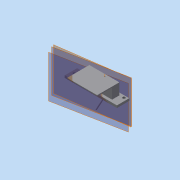
# Autodesk Inventor part: 00_TI_DLP_2000_Chip
Saved by Autodesk Inventor 2019.4 (Build 234330000, 330)
## iProperties
Created: 2019-08-06
Part Number: 00_TI_DLP_2000_Chip
Material: Generic
Document SubType Name: Modeling
Designer: diederichbenedict
Density: 1 g/cm^3
Appearance: Default
Author: diederichbenedict
Autodesk Inventor part; units mm, degrees
ref_plane "YZ Plane" through (0, 0, 0) normal (1, 0, 0) x (0, 1, 0)
ref_plane "XZ Plane" through (0, 0, 0) normal (0, 1, 0) x (-1, 0, 0)
ref_plane "XY Plane" through (0, 0, 0) normal (0, 0, 1) x (1, 0, 0)
sketch "Sketch1" plane through (0, 0, 0) normal (0, 1, 0) x (-1, 0, 0)
  line L0 (14.75, 3.5) -> (-14.75, 3.5)
  line L1 (-14.75, 3.5) -> (-14.75, -3.5)
  line L2 (-14.75, -3.5) -> (14.75, -3.5)
  line L3 (14.75, -3.5) -> (14.75, 3.5)
  line L4 (14.75, 3.5) -> (-14.75, -3.5) construction
  line L5 (-14.75, 3.5) -> (14.75, -3.5) construction
  circle A0 centre (-13, -2.25) radius 0.75
  circle A1 centre (13, -0.25) radius 0.75
  point P0 (0, 0)
  dimension "d0" = 29.5
  dimension "d1" = 7
  dimension "d2" = 1.5
  dimension "d3" = 1.5
  dimension "d4" = 5.75
  dimension "d5" = 3.75
  dimension "d6" = 1.75
  dimension "d7" = 1.75
  constraints: 12 end point, 2 centre point, 2 midpoint, 2 parallel, 1 horizontal, 1 perpendicular
  measures "d0" distance of L2.end L1.end
  measures "d1" distance of L1.end L0.end
  measures "d2" diameter of A0
  measures "d3" diameter of A1
  measures "d4" distance from line of A0.centre L0
  measures "d5" distance from line of A1.centre L0
  measures "d6" distance from line of A1.centre L3
  measures "d7" distance from line of L1 A0.centre
extrude "Extrusion1" add sketch "Sketch1" along normal blind 1.3
sketch "Sketch2" plane through (0, 0, 0) normal (0, -1, 0) x (1, 0, 0)
  line L0 (-3.64, 1.57) -> (10.48, 1.57)
  line L1 (10.48, 1.57) -> (10.48, -3.4)
  line L2 (10.48, -3.4) -> (-3.64, -3.4)
  line L3 (-3.64, -3.4) -> (-3.64, 1.57)
  line L4 (14.75, 3.5) -> (14.75, -3.5) projected
  line L5 (-14.75, -3.5) -> (-14.75, 3.5) projected
  line L6 (14.75, -3.5) -> (-14.75, -3.5) projected
  line L7 (-3.64, 0.335) -> (-2.84, 0.335)
  line L8 (-2.84, 0.335) -> (-2.84, -2.165)
  line L9 (-2.84, -2.165) -> (-3.64, -2.165)
  line L10 (-3.64, -2.165) -> (-3.64, 0.335)
  line L11 (10.48, 0.7644) -> (9.304, -0.4116)
  line L12 (10.48, 0.7644) -> (12.1431, 0.7644) construction
  line L13 (9.304, -0.4116) -> (9.304, -1.4116)
  line L14 (10.48, -2.5876) -> (9.304, -1.4116)
  line L15 (10.48, -2.5876) -> (12.1431, -2.5876) construction
  point P0 (0, 0)
  dimension "d10" = 14.12
  dimension "d11" = 4.97
  dimension "d13" = 11.11
  dimension "d14" = 0.1
  dimension "d15" = 2.5
  dimension "d16" = 0.8
  dimension "d17" = 1.235
  dimension "d18" = 135
  dimension "d19" = 135
  dimension "d20" = 1.176
  dimension "d21" = 1
  constraints: 26 end point, 4 horizontal, 4 parallel, 3 point on line, 2 equal length, 2 perpendicular, 1 vertical
  measures "d10" distance between parallel lines of L1 L3
  measures "d11" distance between parallel lines of L2 L0
  measures "d13" distance between parallel lines of L5 L3
  measures "d14" distance between parallel lines of L2 L6
  measures "d15" distance between parallel lines of L7 L9
  measures "d16" distance between parallel lines of L3 L8
  measures "d17" distance between parallel lines of L7 L0
  measures "d18" angle of L11 L12
  measures "d19" angle of L15 L14
  measures "d20" distance between parallel lines of L13 L1
  measures "d21" distance of L13.end L11.end
extrude "Extrusion2" add sketch "Sketch2" along normal blind 1.2 contours L0 L1 L11 L13 L14 L2 L3 L9 L8 L7
sketch "Sketch3" plane through (0, -1.2, 0) normal (0, -1, 0) x (1, 0, 0)
  line L0 (0.795, 0.57) -> (6.045, 0.57)
  line L1 (6.045, 0.57) -> (6.045, -2.43)
  line L2 (6.045, -2.43) -> (0.795, -2.43)
  line L3 (0.795, -2.43) -> (0.795, 0.57)
  line L4 (0.795, 0.57) -> (6.045, -2.43) construction
  line L5 (6.045, 0.57) -> (0.795, -2.43) construction
  line L6 (-3.64, 1.57) -> (-3.64, 0.335) construction
  line L7 (10.48, 1.57) -> (-3.64, 1.57) construction
  point P0 (0, 0)
  point P1 (3.42, -0.93)
  dimension "d24" = 5.25
  dimension "d25" = 3
  dimension "d26" = 7.06
  dimension "d27" = 2.5
  constraints: 12 end point, 2 parallel, 1 horizontal, 1 midpoint, 1 perpendicular
  measures "d24" distance of L1.end L2.end
  measures "d25" distance of L0.end L1.end
  measures "d26" distance from line of point (3.42, -0.93) L6
  measures "d27" distance from line of point (3.42, -0.93) L7
extrude "Extrusion3" add sketch "Sketch3" along normal blind 1.5
sketch "Sketch4" plane through (0, -1.2, 0) normal (0, -1, 0) x (1, 0, 0)
  line L0 (6.045, 0.57) -> (0.795, 0.57) projected
  line L1 (0.795, 0.57) -> (0.795, -2.43) projected
  line L2 (0.795, -2.43) -> (6.045, -2.43) projected
  line L3 (6.045, -2.43) -> (6.045, 0.57) projected
  line L4 (-1.7742, 0.9523) -> (8.6142, 0.9523)
  line L5 (8.6142, 0.9523) -> (8.6142, -2.8123)
  line L6 (8.6142, -2.8123) -> (-1.7742, -2.8123)
  line L7 (-1.7742, -2.8123) -> (-1.7742, 0.9523)
  line L8 (-1.7742, 0.9523) -> (8.6142, -2.8123) construction
  line L9 (8.6142, 0.9523) -> (-1.7742, -2.8123) construction
  point P0 (0, 0)
  point P1 (3.42, -0.93)
  constraints: 12 end point, 2 midpoint, 2 parallel, 1 horizontal, 1 perpendicular
extrude "Extrusion4" add sketch "Sketch4" along normal blind 1
chamfer "Chamfer1" distance 1 angle 45 4 edges at (3.42, -2.2, -2.8123) (8.6142, -2.2, -0.93) (3.42, -2.2, 0.9523) (-1.7742, -2.2, -0.93)
sketch "Sketch5" plane through (0, -2.7, 0) normal (0, -1, 0) x (1, 0, 0)
  line L0 (6.045, 0.57) -> (0.795, 0.57) projected
  line L1 (0.795, 0.57) -> (0.795, -2.43) projected
  line L2 (0.795, -2.43) -> (6.045, -2.43) projected
  line L3 (6.045, -2.43) -> (6.045, 0.57) projected
  circle A0 centre (3.42, -0.93) radius 0.2753
  point P0 (0, 0)
  constraints: 1 centre point
extrude "Extrusion5" cut sketch "Sketch5" against normal blind 1.5 contours A0
sketch "Sketch6" plane through (0, 1.3, 0) normal (0, 1, 0) x (1, 0, 0)
  circle A0 centre (-13, 0.25) radius 0.75 projected
  circle A1 centre (13, 2.25) radius 0.75 projected
  line L0 (-14.75, -3.5) -> (14.75, -3.5) projected
  line L1 (14.75, -3.5) -> (14.75, 3.5) projected
  line L2 (14.75, 3.5) -> (-14.75, 3.5) projected
  line L3 (-14.75, 3.5) -> (-14.75, -3.5) projected
  line L4 (-6.45, 2.1) -> (10.55, 2.1)
  line L5 (10.55, 2.1) -> (10.55, -2.04)
  line L6 (10.55, -2.04) -> (-6.45, -2.04)
  line L7 (-6.45, -2.04) -> (-6.45, 2.1)
  line L8 (-6.45, 2.1) -> (10.55, -2.04) construction
  line L9 (10.55, 2.1) -> (-6.45, -2.04) construction
  point P0 (0, 0)
  point P1 (2.05, 0.03)
  dimension "d37" = 17
  dimension "d38" = 4.14
  dimension "d39" = 4.2
  dimension "d40" = 1.4
  constraints: 12 end point, 2 midpoint, 2 parallel, 1 horizontal, 1 perpendicular
  measures "d37" distance of L5.end L6.end
  measures "d38" distance of L4.end L5.end
  measures "d39" distance between parallel lines of L5 L1
  measures "d40" distance between parallel lines of L4 L2
extrude "Extrusion6" add sketch "Sketch6" along normal blind 5.9 contours L4 L5 L6 L7
sketch "Sketch7" plane through (0, 7.2, 0) normal (0, 1, 0) x (1, 0, 0)
  circle A0 centre (3.42, 0.93) radius 0.2753 projected
  line L0 (10.55, 2.1) -> (-6.45, 2.1) projected
  line L1 (-6.45, 2.1) -> (-6.45, -2.04) projected
  line L2 (-6.45, -2.04) -> (10.55, -2.04) projected
  line L3 (10.55, -2.04) -> (10.55, 2.1) projected
  line L4 (-6.45, -2.04) -> (10.55, -2.04)
  line L5 (10.55, 2.1) -> (-6.45, 2.1) projected
  line L6 (-6.45, 2.1) -> (10.55, 2.1)
  line L7 (10.55, 2.1) -> (10.55, -10.4875)
  line L8 (10.55, -10.4875) -> (-6.45, -10.4875)
  line L9 (-6.45, -10.4875) -> (-6.45, 2.1)
  point P0 (0, 0)
  point P1 (-2.84, -0.335)
  constraints: 10 end point, 2 horizontal, 2 parallel, 1 perpendicular
extrude "Extrusion7" add sketch "Sketch7" along normal blind 0.5
ref_plane "Work Plane5" through (3.42, -2.7, -0.93) normal (-0.3044173, -0.9025853, 0.3044173) x (0.7071068, 0, 0.7071068)
ref_plane "Work Plane4" through (9.304, -1.2, -0.4116) normal (-0.3044173, -0.9025853, 0.3044173) x (0.7071068, 0, 0.7071068)
sketch "Sketch8" plane through (3.42, -2.7, -0.93) normal (-0.3044173, -0.9025853, 0.3044173) x (0.7071068, 0, 0.7071068)
  circle A0 centre (0, 0) radius 0.2753
  ellipse E0 centre (0, 0) end of major axis (0.2753, 0) minor radius 0.2485 projected
  point P0 (-1.7607, 3.9387)
  constraints: 1 centre point, 2 other
extrude "Extrusion8" cut sketch "Sketch8" against normal blind 10
ref_plane "Work Plane6" through (9.304, -1.2, -0.4116) normal (0.3319665, 0.8829476, -0.3319665) x (0.7071068, 0, 0.7071068)
sketch "Sketch9" plane through (9.304, -1.2, -0.4116) normal (0.3319665, 0.8829476, -0.3319665) x (0.7071068, 0, 0.7071068)
  ellipse E0 centre (-4.5272, -2.6458) end of major axis (-4.2519, -2.6458) minor radius 0.2431 (-4.8024, -2.6458) -> (-4.2519, -2.6458) ccw projected
  ellipse E1 centre (-4.5272, -2.8391) end of major axis (-4.8024, -2.8391) minor radius 0.2693 (-4.2526, -2.8202) -> (-4.5744, -3.1044) ccw projected
  circle A0 centre (-4.5272, -2.8391) radius 0.2753
  point P0 (-6.2879, -6.6292)
  constraints: 1 centre point, 1 coincident, 3 other
extrude "Extrusion9" add sketch "Sketch9" against normal blind 10
body "Solid1"
